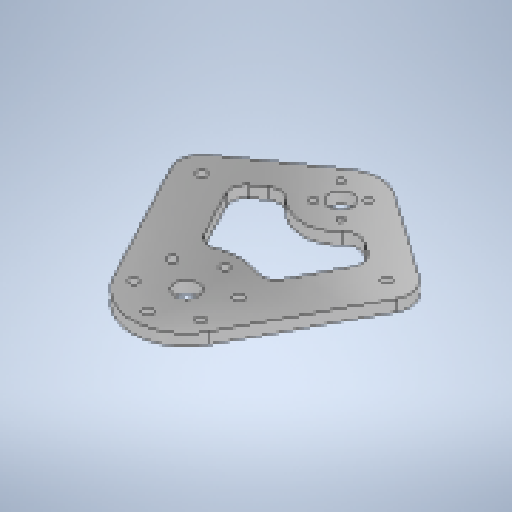
# Autodesk Inventor part: Upright - Bottom
Saved by Autodesk Inventor 2023.4 (Build 274418000, 418)
## iProperties
Created: 2024-09-12
Part Number: Upright - Bottom
Material: Aluminum 6061
Document SubType Name: Modeling
Designer: Nathan Cai
Mass: 41.5661 g
Surface Area: 85.6405 cm^2
Volume: 15.3949 cm^3
Density: 2.7 g/cm^3
Appearance: Aluminum - Flat
Author: Nathan Cai
Autodesk Inventor part; units mm, degrees
ref_plane "YZ Plane" through (0, 0, 0) normal (1, 0, 0) x (0, 1, 0)
ref_plane "XZ Plane" through (0, 0, 0) normal (0, 1, 0) x (-1, 0, 0)
ref_plane "XY Plane" through (0, 0, 0) normal (0, 0, 1) x (1, 0, 0)
sketch "Sketch1" plane through (0, 0, 0) normal (0, 1, 0) x (-1, 0, 0)
  circle A0 centre (0, 0) radius 38.1 construction
  line L0 (0, 0) -> (38.1, 0) construction
  line L1 (0, 0) -> (-38.1, 0) construction
  circle A1 centre (38.1, 0) radius 1.905
  circle A2 centre (-38.1, 0) radius 1.905
  circle A3 centre (38.1, 0) radius 9.525
  circle A4 centre (-38.1, 0) radius 9.525
  line L2 (0, 0) -> (0, 44.45) construction
  circle A5 centre (0, 44.45) radius 76.2 construction
  circle A6 centre (0, 44.45) radius 19.05 construction
  circle A7 centre (0, 0) radius 25.4 construction
  circle A8 centre (0, 44.45) radius 4.7625
  circle A9 centre (0, 44.45) radius 22.225
  line L3 (19.6103, 54.9088) -> (46.5044, 4.4824)
  line L4 (-19.6103, 54.9088) -> (-46.5044, 4.4824)
  line L5 (13.153, 26.535) -> (29.6956, -4.4824)
  line L6 (-13.153, 26.535) -> (-29.6956, -4.4824)
  circle A10 centre (0, 44.45) radius 15.875 construction
  circle A11 centre (0, 60.325) radius 1.905
  circle A12 centre (-13.7482, 52.3875) radius 1.905
  circle A13 centre (-13.7482, 36.5125) radius 1.905
  circle A14 centre (0, 28.575) radius 1.905
  circle A15 centre (13.7482, 36.5125) radius 1.905
  circle A16 centre (13.7482, 52.3875) radius 1.905
  circle A17 centre (0, -19.05) radius 4.7625
  circle A18 centre (0, -19.05) radius 8 construction
  circle A19 centre (0, -19.05) radius 9.5 construction
  line L7 (0, -19.05) -> (9.5, -19.05) construction
  line L8 (0, -19.05) -> (6.7175, -12.3325) construction
  circle A20 centre (5.6569, -13.3931) radius 1.5
  line L9 (0, -19.05) -> (6.7175, -25.7675) construction
  circle A21 centre (6.7175, -25.7675) radius 1.5
  circle A22 centre (-6.7175, -12.3325) radius 1.5
  circle A23 centre (-5.6569, -24.7069) radius 1.5
  circle A24 centre (0, -19.05) radius 15.875
  line L10 (9.1369, -32.032) -> (43.5821, -7.7892)
  line L11 (14.5471, -12.6942) -> (28.7456, -2.7012)
  line L12 (-9.1369, -32.032) -> (-43.5821, -7.7892)
  line L13 (-14.5471, -12.6942) -> (-28.7456, -2.7012)
  point P0 (-29.6956, -4.4824)
  point P1 (29.6956, -4.4824)
  dimension "d14" = 31.75
  dimension "d22" = 16
  dimension "d0" = 76.2
  dimension "d1" = 3.81
  dimension "d2" = 3.81
  dimension "d3" = 19.05
  dimension "d4" = 19.05
  dimension "d5" = 152.4
  dimension "d6" = 38.1
  dimension "d7" = 50.8
  dimension "d8" = 9.525
  dimension "d9" = 44.45
  dimension "d10" = 19.05
  dimension "d15" = 3.81
  dimension "d18" = 360
  dimension "d20" = 9.525
  dimension "d21" = 63.5
  dimension "d23" = 19
  dimension "d24" = 45
  dimension "d25" = 3
  dimension "d26" = 3
  dimension "d29" = 360
  dimension "d31" = 31.75
  dimension "d32" = 12.7
  constraints: 28 end point, 23 centre point, 14 coincident, 11 point on circle, 8 symmetric about line, 5 point on line, 5 tangent, 2 horizontal, 2 parallel, 1 perpendicular, 1 vertical, 1 vertical alignment, 27 other
  measures "d0" diameter of A0
  measures "d1" diameter of A1
  measures "d2" diameter of A2
  measures "d3" diameter of A3
  measures "d4" diameter of A4
  measures "d5" diameter of A5
  measures "d6" diameter of A6
  measures "d7" diameter of A7
  measures "d8" diameter of A8
  measures "d9" diameter of A9
  measures "d10" distance between parallel lines of L3 L5
  measures "d15" diameter of A11
  measures "d20" diameter of A17
  measures "d21" distance of A6.centre A17.centre
  measures "d23" diameter of A19
  measures "d24" angle of L7 L8
  measures "d25" diameter of A20
  measures "d26" diameter of A21
  measures "d31" diameter of A24
  measures "d32" distance between parallel lines of L10 L11
extrude "Extrusion1" add sketch "Sketch1" along normal blind 4.7625 contours A3 | A3 L5 A9 L3 | L10 A24 L11 L5 A3 | A9 | A24 | A9 L6 A4 L4 | L12 A4 L6 L13 A24 | A4
fillet "Fillet1" radius 6.35 6 edges at (-13.153, 2.3813, 26.535) (13.153, 2.3813, 26.535) (-14.5471, 2.3813, -12.6942) (-28.7456, 2.3813, -2.7012) (14.5471, 2.3813, -12.6942) (28.7456, 2.3813, -2.7012)
equation "\"d2\" = d1"
equation "\"d4\" = d3"
body "Solid1"
